Autodesk Fusion 360 part; units mm, degrees
(part 3 of 5)
sketch "Sketch6 (3)" plane through (0, 18.9, 0) normal (0, -1, 0) x (1, 0, 0) in component "main-switchbody (3)"
  line L0 (13.95, 0) -> (16.95, 0)
  line L1 (16.95, 0) -> (16.95, 6)
  line L2 (16.95, 6) -> (13.95, 6)
  line L3 (13.95, 6) -> (13.95, 0)
  line L4 (13.95, 6) -> (13.95, 4.5) construction
  line L5 (16.95, 6) -> (16.95, 4.5) construction
  arc A0 (16.95, 4.5) -> (13.95, 4.5) centre (15.45, 4.5) ccw
  constraint coincident L2.end L3.start
  constraint coincident L3 L4.end
  constraint perpendicular L2 L4
  constraint coincident L1.end L2.start
  constraint coincident L1 L5.end
  constraint perpendicular L2 L5
  constraint tangent L2 A0
extrude "Extrude10''" cut sketch "Sketch6 (3)" against normal blind 1.1 contours L2 L3 A0 | L1 L2 A0 bodies 24 in component "main-switchbody (3)"
sketch "Sketch7 (3)" plane through (0, 0, 4) normal (0, 0, 1) x (-1, 0, 0) in component "main-switchbody (3)"
  line L0 (-3.05, -16.95) -> (-16.95, -16.95)
  line L1 (-16.95, -16.95) -> (-16.95, -3.05)
  line L2 (-16.95, -3.05) -> (-3.05, -3.05)
  line L3 (-3.05, -3.05) -> (-3.05, -16.95)
  line L4 (-6.05, -20) -> (-6.05, -18.9)
  line L5 (-6.05, -18.9) -> (-3.05, -18.9)
  line L6 (-3.05, -18.9) -> (-3.05, -20)
  line L7 (-3.05, -20) -> (0, -20)
  line L8 (0, -20) -> (0, 0)
  line L9 (0, 0) -> (-3.05, 0)
  line L10 (-3.05, 0) -> (-3.05, -1.1)
  line L11 (-3.05, -1.1) -> (-6.05, -1.1)
  line L12 (-6.05, -1.1) -> (-6.05, 0)
  line L13 (-6.05, 0) -> (-13.95, 0)
  line L14 (-13.95, 0) -> (-13.95, -1.1)
  line L15 (-13.95, -1.1) -> (-16.95, -1.1)
  line L16 (-16.95, -1.1) -> (-16.95, 0)
  line L17 (-16.95, 0) -> (-20, 0)
  line L18 (-20, 0) -> (-20, -20)
  line L19 (-20, -20) -> (-16.95, -20)
  line L20 (-16.95, -20) -> (-16.95, -18.9)
  line L21 (-16.95, -18.9) -> (-13.95, -18.9)
  line L22 (-13.95, -18.9) -> (-13.95, -20)
  line L23 (-13.95, -20) -> (-6.05, -20)
  line L24 (-20, -10) -> (-20, -11.5) construction
  line L25 (-20, -10) -> (-20, -8.5) construction
  line L26 (-20, -8.5) -> (-19, -8.5) construction
  line L27 (-19, -8.5) -> (-19, -11.5) construction
  line L28 (-19, -11.5) -> (-20, -11.5) construction
  line L29 (-20, -11.5) -> (-21, -11.5) construction
  line L30 (-21, -11.5) -> (-21, -8.5) construction
  line L31 (-21, -8.5) -> (-20, -8.5) construction
  line L32 (-19, -11.5) -> (-21, -11.5)
  line L33 (-21, -11.5) -> (-21, -8.5)
  line L34 (-21, -8.5) -> (-19, -8.5)
  line L35 (-19, -8.5) -> (-19, -11.5)
  dimension "d41_6" = 1.5
  dimension "d42_6" = 1
  constraint midpoint L18 L24.start
  constraint parallel L18 L24
  constraint coincident L18 L25.end
  constraint parallel L18 L25
  constraint perpendicular L25 L26
  constraint perpendicular L26 L27
  constraint perpendicular L24 L29
  constraint perpendicular L29 L30
  constraint horizontal L32
  constraint vertical L33
  constraint horizontal L34
  constraint vertical L35
  measures "d41_6" distance of L24.start L24.end
  measures "d42_6" distance of L24.end L29.end
extrude "Extrude11''" add sketch "Sketch7 (3)" along normal blind 3 contours L18 L32 L33 L34 | L18 L32 L34 L35 bodies 20 in component "main-switchbody (3)"
extrude "Extrude12''" add 1 faces at (20, 8.5, 6) along direction (0, -1, 0) blind 0.5 on bodies 20 bodies 20 in component "main-switchbody (3)"
extrude "Extrude13''" add 1 faces at (20, 11.5, 6) along direction (0, 1, 0) blind 0.5 on bodies 20 bodies 20 in component "main-switchbody (3)"
extrude "Extrude14''" add 1 faces at (20.3333, 10.6667, 7) along direction (0, 0, 1) blind 0.75 on bodies 20 bodies 20 in component "main-switchbody (3)"
sketch "Sketch8 (3)" plane through (0, 0, 4) normal (0, 0, -1) x (1, 0, 0) in component "main-switchbody (3)"
  line L0 (20, -8) -> (20, -12)
  line L1 (20, -12) -> (21, -12)
  line L2 (21, -12) -> (21, -8)
  line L3 (21, -8) -> (20, -8)
  line L4 (20, -12) -> (20, -8)
  constraint coincident L0.end L1.start
  constraint coincident L0.start L3.end
extrude "Extrude15''" add sketch "Sketch8 (3)" along normal blind 2 bodies 20 in component "main-switchbody (3)"
sketch "Sketch9 (5)" plane through (19, 0, 0) normal (-1, 0, 0) x (0, -1, 0) in component "main-switchbody (3)"
  line L0 (-12, 4) -> (-8, 4)
  line L1 (-8, 4) -> (-8, 7.75)
  line L2 (-8, 7.75) -> (-12, 7.75)
  line L3 (-12, 7.75) -> (-12, 4)
  line L4 (-12, 7.75) -> (-12, 5.75) construction
  line L5 (-12, 5.75) -> (-8, 5.75) construction
  line L6 (-12, 7.75) -> (-8, 7.75)
  line L7 (-8, 7.75) -> (-8, 5.75)
  line L8 (-8, 5.75) -> (-12, 5.75)
  line L9 (-12, 5.75) -> (-12, 7.75)
  dimension "d53_6" = 2
  constraint coincident L2.end L3.start
  constraint perpendicular L2 L4
  constraint coincident L1 L5.end
  constraint perpendicular L1 L5
  constraint horizontal L6
  constraint vertical L7
  constraint horizontal L8
  constraint vertical L9
  measures "d53_6" distance of L2.end L4.end
extrude "Extrude16''" add sketch "Sketch9 (5)" along normal blind 0.5 contours L1 L2 L3 L6 L7 L8 L9 bodies 20 in component "main-switchbody (3)"
extrude "Extrude17''" cut 1 faces at (2.1, 9.3333, 6.9167) along direction (-1, 0, 0) blind 0.3 on bodies 19 bodies 19 in component "main-switchbody (3)"
extrude "Extrude18''" cut sketch "Sketch1 (13)" along normal blind 2.7 contours L44 L84 L85 L86 L87 bodies 20 in component "main-switchbody (3)"
extrude "Extrude19''" cut sketch "Sketch1 (13)" along normal blind 2.7 contours L46 L80 L81 L82 L83 bodies 20 in component "main-switchbody (3)"
extrude "Extrude20''" add sketch "Sketch1 (13)" against normal blind 0.2 contours L39 L40 L41 L42 L47 L48 L50 L51 L52 L54 L56 L57 L58 L60 L61 L62 L63 L64 L65 L66 L67 L68 | L39 L59 L60 L61 L62 | L42 L63 L64 L65 L66 L67 L68 | L39 L55 L56 L57 L58 | L41 L47 L48 L49 L50 | L41 L51 L52 L53 L54 bodies 19 20 21 22 23 24 in component "main-switchbody (3)"
fillet "Fillet1''" radius 1 2 edges at (21, 10, 7.75) (-0.9, 10, 7.5) on bodies 19 20 in component "main-switchbody (3)"
extrude "Extrude21''" add 1 faces at (2.8833, 9.1667, 2.7) along direction (0, 0, -1) blind 2.9 on bodies 19 bodies 19 in component "main-switchbody (3)"
extrude "Extrude22''" add 1 faces at (17.1167, 10.8333, 2.7) along direction (0, 0, -1) blind 2.9 on bodies 19 bodies 19 in component "main-switchbody (3)"
sketch "Sketch10 (3)" plane through (0, 0, 4) normal (0, 0, 1) x (-1, 0, 0) in component "main-switchbody (3)"
  line L0 (-3.05, -16.95) -> (-16.95, -16.95)
  line L1 (-16.95, -16.95) -> (-16.95, -3.05)
  line L2 (-16.95, -3.05) -> (-3.05, -3.05)
  line L3 (-3.05, -3.05) -> (-3.05, -16.95)
  line L4 (0, -12) -> (-1.1, -12)
  line L5 (-1.1, -12) -> (-1.1, -8)
  line L6 (-1.1, -8) -> (0, -8)
  line L7 (0, -8) -> (0, 0)
  line L8 (0, 0) -> (-3.05, 0)
  line L9 (-3.05, 0) -> (-3.05, -1.1)
  line L10 (-3.05, -1.1) -> (-6.05, -1.1)
  line L11 (-6.05, -1.1) -> (-6.05, 0)
  line L12 (-6.05, 0) -> (-13.95, 0)
  line L13 (-13.95, 0) -> (-13.95, -1.1)
  line L14 (-13.95, -1.1) -> (-16.95, -1.1)
  line L15 (-16.95, -1.1) -> (-16.95, 0)
  line L16 (-16.95, 0) -> (-20, 0)
  line L17 (-20, 0) -> (-20, -8)
  line L18 (-20, -8) -> (-19, -8)
  line L19 (-19, -8) -> (-19, -12)
  line L20 (-19, -12) -> (-20, -12)
  line L21 (-20, -12) -> (-20, -20)
  line L22 (-20, -20) -> (-16.95, -20)
  line L23 (-16.95, -20) -> (-16.95, -18.9)
  line L24 (-16.95, -18.9) -> (-13.95, -18.9)
  line L25 (-13.95, -18.9) -> (-13.95, -20)
  line L26 (-13.95, -20) -> (-6.05, -20)
  line L27 (-6.05, -20) -> (-6.05, -18.9)
  line L28 (-6.05, -18.9) -> (-3.05, -18.9)
  line L29 (-3.05, -18.9) -> (-3.05, -20)
  line L30 (-3.05, -20) -> (0, -20)
  line L31 (0, -20) -> (0, -12)
  line L32 (-3.05, -10) -> (-3.05, -12.5) construction
  line L33 (-3.05, -12.5) -> (-3.05, -7.5) construction
  line L34 (-3.05, -7.5) -> (-2.55, -7.5) construction
  line L35 (-2.55, -7.5) -> (-3.05, -7.5) construction
  line L36 (-3.05, -7.5) -> (-3.05, -12.5) construction
  line L37 (-3.05, -12.5) -> (-2.55, -12.5) construction
  line L38 (-2.55, -12.5) -> (-2.55, -7.5) construction
  line L39 (-3.05, -12.5) -> (-16.95, -12.5) construction
  line L40 (-16.95, -12.5) -> (-16.95, -7.5) construction
  line L41 (-16.95, -7.5) -> (-17.45, -7.5) construction
  line L42 (-17.45, -7.5) -> (-16.95, -7.5) construction
  line L43 (-16.95, -7.5) -> (-16.95, -12.5) construction
  line L44 (-16.95, -12.5) -> (-17.45, -12.5) construction
  line L45 (-17.45, -12.5) -> (-17.45, -7.5) construction
  line L46 (-16.95, -12.5) -> (-17.45, -12.5)
  line L47 (-17.45, -12.5) -> (-17.45, -7.5)
  line L48 (-17.45, -7.5) -> (-16.95, -7.5)
  line L49 (-16.95, -7.5) -> (-16.95, -12.5)
  line L50 (-2.55, -12.5) -> (-3.05, -12.5)
  line L51 (-3.05, -12.5) -> (-3.05, -7.5)
  line L52 (-3.05, -7.5) -> (-2.55, -7.5)
  line L53 (-2.55, -7.5) -> (-2.55, -12.5)
  dimension "d75_3" = 5
  dimension "d76_3" = 0.5
  dimension "d77_3" = 0.5
  constraint midpoint L3 L32.start
  constraint coincident L3 L32.end
  constraint perpendicular L0 L32
  constraint parallel L3 L33
  constraint perpendicular L33 L34
  constraint horizontal L35
  constraint vertical L36
  constraint horizontal L37
  constraint vertical L38
  constraint coincident L1 L39.end
  constraint perpendicular L1 L39
  constraint coincident L1 L40.end
  constraint perpendicular L39 L40
  constraint perpendicular L40 L41
  constraint horizontal L42
  constraint vertical L43
  constraint horizontal L44
  constraint vertical L45
  constraint horizontal L46
  constraint vertical L47
  constraint horizontal L48
  constraint vertical L49
  constraint horizontal L50
  constraint vertical L51
  constraint horizontal L52
  constraint vertical L53
  measures "d75_3" distance of L32.end L33.end
  measures "d76_3" distance of L33.end L34.end
  measures "d77_3" distance of L40.end L41.end
extrude "Extrude23''" cut sketch "Sketch10 (3)" against normal blind 2.9 contours L3 L50 L51 L52 L53 | L1 L46 L47 L48 L49 bodies 19 in component "main-switchbody (3)"
extrude "Extrude24''" cut 2 faces at (4.8122, 18.9, 5.1079) (15.1626, 18.9, 5.4316) along direction (0, 1, 0) blind 0.25 on bodies 19 bodies 19 in component "main-switchbody (3)"
extrude "Extrude25''" cut 2 faces at (4.2822, 1.1, 5.1824) (15.2673, 1.1, 4.9654) along direction (0, -1, 0) blind 0.25 on bodies 19 bodies 19 in component "main-switchbody (3)"
extrude "Extrude26''" add 1 faces at (1.0167, 12.3167, -0.2) along direction (0, 0, -1) blind 1 on bodies 19 bodies 19 in component "main-switchbody (3)"
extrude "Extrude27''" cut 1 faces at (1.0167, 12.3167, -1.2) along direction (0, 0, 1) blind 0.2 on bodies 19 bodies 19 in component "main-switchbody (3)"
extrude "Extrude28''" cut 2 faces at (17.1167, 10.8333, 1.1) (2.8833, 9.1667, 1.1) along direction (0, 0, -1) blind 0.8 on bodies 19 bodies 19 in component "main-switchbody (3)"
extrude "Extrude29''" cut 1 faces at (18.8333, 9.3333, 5.75) along direction (0, 0, 1) blind 0.2 on bodies 19 bodies 19 in component "main-switchbody (3)"
extrude "Extrude30''" cut 1 faces at (1.3333, 10.6667, 5.75) along direction (0, 0, 1) blind 0.2 on bodies 19 bodies 19 in component "main-switchbody (3)"
sketch "Sketch1 (14)" plane through (0, 0, 0.0152) normal (0, 0, -1) x (1, 0, 0) in component "mxledbit-switchbody v10 (3)"
  line L0 (4.5419, -16.2374) -> (4.5419, -2.3374)
  line L1 (4.5419, -2.3374) -> (18.4419, -2.3374)
  line L2 (18.4419, -2.3374) -> (18.4419, -16.2374)
  line L3 (18.4419, -16.2374) -> (4.5419, -16.2374)
  line L4 (1.4919, -19.2874) -> (21.4919, -19.2874)
  line L5 (21.4919, -19.2874) -> (21.4919, 0.7126)
  line L6 (21.4919, 0.7126) -> (1.4919, 0.7126)
  line L7 (1.4919, 0.7126) -> (1.4919, -19.2874)
ref_plane "WorkPlane1" through (5, 36.1899, 12.0831) normal (0, -0.996195, 0.087156) x (1, 0, 0) in component "wheel (2)"
sketch "Sketch2 (11)" plane through (5, 36.1899, 12.0831) normal (0, -0.996195, 0.087156) x (1, 0, 0) in component "wheel (2)"
  circle A0 centre (0, 0) radius 85
  dimension "d64_3" = 170
  constraint coincident A0.centre origin
  measures "d64_3" diameter of A0
component_pattern "component pattern''" in component "Middle"
sketch "Sketch2 (12)" plane through (0, 32.8735, -2.8761) normal (0, -0.996195, 0.087156) x (1, 0, 0) in component "IND-Sketch (2)"
  circle A0 centre (5, 15.1913) radius 85
  line L0 (5, 15.1913) -> (5, -69.8087) construction
  line L1 (5, -69.8087) -> (-12, -69.8087) construction
  line L2 (-12, -69.8087) -> (22, -69.8087)
  line L3 (22, -69.8087) -> (22, 15.1913)
  line L4 (22, 15.1913) -> (-12, 15.1913)
  line L5 (-12, 15.1913) -> (-12, -69.8087)
  dimension "d69_3" = 85
  dimension "d70_3" = 17
  dimension "d71_3" = 34
  dimension "d72_3" = 85
  constraint coincident A0.centre L0.start
  constraint vertical L0
  constraint perpendicular L0 L1
  constraint horizontal L2
  constraint vertical L3
  constraint horizontal L4
  constraint vertical L5
  measures "d69_3" distance of A0.centre L0.end
  measures "d70_3" distance of L0.end L1.end
  measures "d71_3" distance of L1.end L2.end
  measures "d72_3" distance of L1.end L4.end
sketch "Sketch9 (6)" plane through (5, 41.9534, 55.6343) normal (0, 0.573576, 0.819152) x (-1, 0, 0) in component "IND-Sketch (2)"
  line L0 (-45, -9.823) -> (5, -9.823) construction
  line L1 (-20, -9.823) -> (5, -9.823) construction
  line L2 (-20, -9.823) -> (-45, -9.823) construction
  circle A0 centre (-20, -9.823) radius 75 construction
  point P0 (-20, -9.823)
  point P1 (-45, -9.823)
  point P2 (5, -9.823)
  point P3 (5, -9.823)
  point P4 (-45, -9.823)
  dimension "d38_3" = 34
  dimension "d39_3" = 17
  dimension "d40_3" = 17
  dimension "d41_3" = 170
  constraint coincident P4 P1
  constraint horizontal L0
  constraint coincident P0 L1.start
  constraint parallel L0 L1
  constraint parallel L0 L2
sketch "Sketch1 (15)" plane through (0, 54.7581, -45.9475) normal (0, -0.766044, 0.642788) x (1, 0, 0) in component "IND-Sketch (2)"
  line L0 (-1.3269, 70.632) -> (-1.3269, 84.532)
  line L1 (-1.3269, 84.532) -> (12.5731, 84.532)
  line L2 (12.5731, 84.532) -> (12.5731, 70.632)
  line L3 (12.5731, 70.632) -> (-1.3269, 70.632)
  line L4 (-4.3769, 67.582) -> (15.6231, 67.582)
  line L5 (15.6231, 67.582) -> (15.6231, 87.582)
  line L6 (15.6231, 87.582) -> (-4.3769, 87.582)
  line L7 (-4.3769, 87.582) -> (-4.3769, 67.582)
  line L8 (-4.3769, 77.582) -> (15.6231, 77.582) construction
  line L9 (5.6231, 87.582) -> (5.6231, 67.582) construction
  point P0 (5.6231, 77.582)
  constraint midpoint L7 L8.start
  constraint midpoint L5 L8.end
  constraint midpoint L6 L9.start
  constraint midpoint L4 L9.end
  constraint midpoint L8 P0
ref_plane "WorkPlane2" through (0, 49, 0) normal (0, 1, 0) x (0, 0, 1) in component "IND-Sketch (3)"
sketch "IND-originXY (4)" plane through (0, 0, 0) normal (0, 0, 1) x (1, 0, 0) in component "IND-Sketch (3)"
  line L0 (0, 0) -> (0, 16) construction
  line L1 (0, 16) -> (16, 16) construction
  line L2 (16, 16) -> (16, -33) construction
  line L3 (16, -33) -> (-33, -33) construction
  line L4 (0, 16) -> (24.5, 16) construction
  point P0 (24.5, 16)
  dimension "d20_7" = 16
  dimension "d21_7" = 16
  dimension "d29_7" = 49
  dimension "d30_7" = 49
  dimension "d34_7" = 24.5
  constraint coincident L0.start origin
  constraint vertical L0
  constraint perpendicular L0 L1
  constraint perpendicular L1 L2
  constraint perpendicular L0 L3
  constraint perpendicular L0 L4
  constraint coincident P0 L4.end
  measures "d20_7" distance of L0.start L0.end
  measures "d21_7" distance of L0.end L1.end
  measures "d29_7" distance of L1.end L2.end
  measures "d30_7" distance of L2.end L3.end
  measures "d34_7" distance of L0.end P0
sketch "IND-originXZ (4)" plane through (0, 49, 0) normal (0, 1, 0) x (1, 0, 0) in component "IND-Sketch (3)"
  line L0 (0, 0) -> (16, 0) construction
  line L1 (10, 0) -> (10, -10) construction
  line L2 (10, -10) -> (0, -10) construction
  line L3 (0, -10) -> (0, 0) construction
  line L4 (10, -10) -> (5, -10) construction
  line L5 (0, -10) -> (5, -10) construction
  line L6 (0, -10) -> (5, -10) construction
  point P0 (16, 0)
  point P1 (0, -10)
  point P2 (10, -10)
  point P3 (24.5, 0)
  point P4 (5, -10)
  dimension "d26_7" = 10
  dimension "d27_7" = 49
  dimension "d28_7" = 49
  dimension "d36_7" = 24.5
  dimension "d37_7" = 24.5
  constraint coincident P0 L1.start
  constraint perpendicular L0 L1
  constraint perpendicular L1 L2
  constraint coincident L0.start L3.end
  constraint coincident P1 L2.end
  constraint coincident P2 L1.end
  constraint midpoint L2 P4
  constraint perpendicular L1 L4
  constraint parallel L4 L6
  measures "d26_7" distance of L1.start P2
ref_plane "WorkPlane3" through (5, 49, 10) normal (0, 1, 0) x (-1, 0, 0) in component "IND-Sketch (3)"
sketch "IND-path (4)" plane through (5, 49, 10) normal (0, 1, 0) x (-1, 0, 0) in component "IND-Sketch (3)"
  line L0 (-5, 0) -> (5, 0) construction
  line L1 (5, 0) -> (-5, 0) construction
  circle A0 centre (0, 0) radius 75 construction
  line L2 (0, 0) -> (24.5, 0) construction
  line L3 (0, 0) -> (-24.5, 0) construction
  line L4 (0, 0) -> (0, -75) construction
  line L5 (0, -75) -> (6.95, -75) construction
  line L6 (0, -75) -> (-6.95, -75) construction
  point P0 (-5, 0)
  point P1 (5, 0)
  point P2 (0, -75)
  dimension "d32_7" = 150
  dimension "d33_7" = 24.5
  dimension "d35_7" = 24.5
  dimension "d42_7" = 75
  dimension "d43_7" = 6.95
  dimension "d44_7" = 6.95
  dimension "d67_7" = 90
  constraint coincident P1 L0.end
  constraint coincident P0 L0.start
  constraint coincident A0.centre L2.start
  constraint parallel L1 L2
  constraint parallel L0 L3
  constraint coincident P2 L4.end
  constraint perpendicular L4 L5
  constraint perpendicular L4 L6
  measures "d32_7" diameter of A0
  measures "d33_7" distance of A0.centre L2.end
  measures "d35_7" distance of A0.centre L3.end
  measures "d42_7" distance of A0.centre P2
  measures "d43_7" distance of P2 L5.end
  measures "d44_7" distance of P2 L6.end
  measures "d67_7" angle of L2 L4
sketch "Sketch1 (16)" plane through (5, 49, 10) normal (0, 1, 0) x (-1, 0, 0) in component "wheel (3)"
  circle A0 centre (0, 0) radius 75
  line L0 (0, -75) -> (6.95, -75)
  line L1 (0, -75) -> (-6.95, -75)
  line L2 (0, -75) -> (0, 75) construction
  line L3 (0, 0) -> (75, 0) construction
  circle A1 centre (0, 0) radius 75
  point P0 (0, -75)
  dimension "d45_7" = 150
  dimension "d46_7" = 75
  dimension "d47_7" = 150
  constraint coincident P0 L0.start
  constraint perpendicular L0 L2
  constraint coincident A0.centre L3.start
  constraint perpendicular L2 L3
  measures "d45_7" distance of P0 L2.end
  measures "d46_7" distance of A0.centre L3.end
  measures "d47_7" diameter of A1
extrude "Extrude1'''''''''" add sketch "Sketch1 (16)" along normal blind 4 separate body makes body 25 in component "wheel (3)"
ref_plane "WorkPlane1" through (5, 70.3992, -65) normal (0, 0, -1) x (1, 0, 0) in component "plug (3)"
sketch "Sketch1 (17)" plane through (5, 31.3992, -65) normal (0, 0, -1) x (1, 0, 0) in component "plug (3)"
  line L0 (-75, -21.6008) -> (75, -21.6008)
  line L1 (-75, -21.6008) -> (75, -21.6008)
  line L2 (-75, -17.6008) -> (75, -17.6008)
  line L3 (-75, -17.6008) -> (75, -17.6008)
  line L4 (0, -17.6008) -> (0, -21.6008) construction
  line L5 (0, -17.6008) -> (-6.95, -17.6008) construction
  line L6 (0, -17.6008) -> (6.95, -17.6008) construction
  line L7 (6.95, -17.6008) -> (6.95, -21.6008) construction
  line L8 (-6.95, -17.6008) -> (-6.95, -21.6008) construction
  line L9 (-6.95, -21.6008) -> (6.95, -21.6008) construction
  line L10 (6.95, -21.6008) -> (-6.95, -21.6008)
  line L11 (-6.95, -21.6008) -> (-6.95, -17.6008)
  line L12 (-6.95, -17.6008) -> (6.95, -17.6008)
  line L13 (6.95, -17.6008) -> (6.95, -21.6008)
  point P0 (0, -17.6008)
  dimension "d51_7" = 6.95
  dimension "d52_7" = 6.95
  constraint coincident P0 L4.start
  constraint midpoint L1 L4.end
  constraint perpendicular L4 L5
  constraint perpendicular L4 L6
  constraint coincident L1 L7.end
  constraint perpendicular L1 L7
  constraint coincident L0 L8.end
  constraint perpendicular L0 L8
  constraint horizontal L10
  constraint vertical L11
  constraint horizontal L12
  constraint vertical L13
  measures "d51_7" distance of P0 L5.end
  measures "d52_7" distance of P0 L6.end
extrude "Extrude1''''''''''" add sketch "Sketch1 (17)" along normal blind 4 separate body makes body 26 in component "plug (3)"
sketch "Sketch2 (13)" plane through (0, 0, -65) normal (0, 0, 1) x (1, 0, 0) in component "plug (3)"
  line L0 (-1.95, 49) -> (11.95, 49)
  line L1 (11.95, 49) -> (11.95, 53)
  line L2 (11.95, 53) -> (-1.95, 53)
  line L3 (-1.95, 53) -> (-1.95, 49)
extrude "Extrude2''''''" add 1 faces at (2.6833, 53, -67.6667) along direction (0, 1, 0) blind 4.95 on bodies 26 bodies 26 in component "plug (3)"
extrude "Extrude3''''''" add 1 faces at (2.6833, 49, -67.6667) along direction (0, -1, 0) blind 4.95 on bodies 26 bodies 26 in component "plug (3)"
sketch "Sketch1 (18)" plane through (0, 0, 0) normal (0, 0, 1) x (1, 0, 0) in component "main-switchbody (5)"
  line L0 (0, 0) -> (0, 20) construction
  line L1 (0, 20) -> (20, 20) construction
  line L2 (20, 20) -> (20, 0) construction
  line L3 (20, 0) -> (0, 0) construction
  line L4 (0, 0) -> (20, 20) construction
  line L5 (20, 0) -> (0, 20) construction
  line L6 (10, 0) -> (18.9, 0) construction
  line L7 (10, 10) -> (18.9, 10) construction
  line L8 (18.9, 10) -> (18.9, 18.9) construction
  line L9 (18.9, 18.9) -> (1.1, 18.9) construction
  line L10 (1.1, 18.9) -> (1.1, 1.1) construction
  line L11 (1.1, 1.1) -> (18.9, 1.1) construction
  line L12 (18.9, 1.1) -> (18.9, 18.9) construction
  line L13 (10, 10) -> (3.05, 10) construction
  line L14 (3.05, 10) -> (3.05, 16.95) construction
  line L15 (3.05, 16.95) -> (16.95, 16.95) construction
  line L16 (16.95, 16.95) -> (16.95, 3.05) construction
  line L17 (16.95, 3.05) -> (3.05, 3.05) construction
  line L18 (3.05, 3.05) -> (3.05, 16.95) construction
  line L19 (3.05, 3.05) -> (0, 3.05) construction
  line L20 (3.05, 3.05) -> (3.05, 0) construction
  line L21 (16.95, 3.05) -> (20, 3.05) construction
  line L22 (16.95, 16.95) -> (20, 16.95) construction
  line L23 (16.95, 16.95) -> (16.95, 20) construction
  line L24 (3.05, 16.95) -> (3.05, 20) construction
  line L25 (3.05, 16.95) -> (0, 16.95) construction
  line L26 (3.05, 18.9) -> (6.05, 18.9) construction
  line L27 (6.05, 18.9) -> (6.05, 20) construction
  line L28 (16.95, 18.9) -> (13.95, 18.9) construction
  line L29 (13.95, 18.9) -> (13.95, 20) construction
  line L30 (16.95, 3.05) -> (16.95, 0) construction
  line L31 (16.95, 1.1) -> (13.95, 1.1) construction
  line L32 (13.95, 1.1) -> (13.95, 0) construction
  line L33 (3.05, 1.1) -> (6.05, 1.1) construction
  line L34 (6.05, 1.1) -> (6.05, 0) construction
  line L35 (0, 20) -> (20, 20) construction
  line L36 (20, 20) -> (20, 0) construction
  line L37 (20, 0) -> (0, 0) construction
  line L38 (0, 0) -> (0, 20) construction
  line L39 (0, 20) -> (20, 20)
  line L40 (20, 20) -> (20, 0)
  line L41 (20, 0) -> (0, 0)
  line L42 (0, 0) -> (0, 20)
  line L43 (16.95, 3.05) -> (3.05, 3.05)
  line L44 (3.05, 3.05) -> (3.05, 16.95)
  line L45 (3.05, 16.95) -> (16.95, 16.95)
  line L46 (16.95, 16.95) -> (16.95, 3.05)
  line L47 (3.05, 1.1) -> (6.05, 1.1)
  line L48 (6.05, 1.1) -> (6.05, 0)
  line L49 (6.05, 0) -> (3.05, 0)
  line L50 (3.05, 0) -> (3.05, 1.1)
  line L51 (13.95, 1.1) -> (16.95, 1.1)
  line L52 (16.95, 1.1) -> (16.95, 0)
  line L53 (16.95, 0) -> (13.95, 0)
  line L54 (13.95, 0) -> (13.95, 1.1)
  line L55 (13.95, 20) -> (16.95, 20)
  line L56 (16.95, 20) -> (16.95, 18.9)
  line L57 (16.95, 18.9) -> (13.95, 18.9)
  line L58 (13.95, 18.9) -> (13.95, 20)
  line L59 (3.05, 20) -> (6.05, 20)
  line L60 (6.05, 20) -> (6.05, 18.9)
  line L61 (6.05, 18.9) -> (3.05, 18.9)
  line L62 (3.05, 18.9) -> (3.05, 20)
  line L63 (1.1, 10) -> (1.1, 12)
  line L64 (1.1, 10) -> (1.1, 8)
  line L65 (1.1, 8) -> (-1.9, 8)
  line L66 (-1.9, 8) -> (1.1, 8)
  line L67 (1.1, 8) -> (1.1, 12)
  line L68 (1.1, 12) -> (-1.9, 12)
  line L69 (-1.9, 12) -> (-1.9, 8)
  line L70 (3.05, 10) -> (3.05, 7.5) construction
  line L71 (3.05, 7.5) -> (2.55, 7.5) construction
  line L72 (2.55, 7.5) -> (2.55, 12.5) construction
  line L73 (2.55, 12.5) -> (3.05, 12.5085) construction
  line L74 (3.05, 12.5085) -> (3.05, 7.5) construction
  line L75 (2.55, 12.5) -> (16.95, 12.5) construction
  line L76 (16.95, 12.5) -> (17.45, 12.5) construction
  line L77 (17.45, 12.5) -> (17.45, 7.5) construction
  line L78 (17.45, 7.5) -> (16.95, 7.5) construction
  line L79 (16.95, 7.5) -> (16.95, 12.5) construction
  line L80 (17.45, 7.5) -> (16.95, 7.5)
  line L81 (16.95, 7.5) -> (16.95, 12.5)
  line L82 (16.95, 12.5) -> (17.45, 12.5)
  line L83 (17.45, 12.5) -> (17.45, 7.5)
  line L84 (3.05, 7.5) -> (2.55, 7.5)
  line L85 (2.55, 7.5) -> (2.55, 12.5)
  line L86 (2.55, 12.5) -> (3.05, 12.5)
  line L87 (3.05, 12.5) -> (3.05, 7.5)
  dimension "d1_5" = 20
  dimension "d2_5" = 20
  dimension "d3_5" = 8.9
  dimension "d4_5" = 8.9
  dimension "d5_5" = 8.9
  dimension "d6_5" = 17.8
  dimension "d7_5" = 17.8
  dimension "d8_5" = 6.95
  dimension "d9_5" = 6.95
  dimension "d10_5" = 13.9
  dimension "d11_5" = 13.9
  dimension "d12_5" = 13.9
  dimension "d13_5" = 3
  dimension "d14_5" = 3
  dimension "d15_5" = 3
  dimension "d16_5" = 3
  dimension "d21_9" = 3
  dimension "d58_9" = 2.5
  dimension "d59_9" = 0.5
  dimension "d60_9" = 5
  dimension "d61_9" = 0.5
  dimension "d62_9" = 5
  constraint coincident L0.start L3.end
  constraint vertical L0
  constraint perpendicular L0 L1
  constraint perpendicular L1 L2
  constraint perpendicular L0 L3
  constraint midpoint L3 L6.start
  constraint parallel L3 L6
  constraint midpoint L4 L7.start
  constraint parallel L6 L7
  constraint perpendicular L7 L8
  constraint perpendicular L8 L9
  constraint perpendicular L9 L10
  constraint coincident L5 L11.end
  constraint perpendicular L10 L11
  constraint perpendicular L12 L13
  constraint perpendicular L13 L14
  constraint perpendicular L14 L15
  constraint perpendicular L7 L16
  constraint perpendicular L16 L17
  constraint coincident L0 L19.end
  constraint perpendicular L0 L19
  constraint coincident L3 L20.end
  constraint perpendicular L3 L20
  constraint coincident L2 L21.end
  constraint perpendicular L2 L21
  constraint coincident L2 L22.end
  constraint perpendicular L2 L22
  constraint coincident L1 L23.end
  constraint perpendicular L1 L23
  constraint coincident L1 L24.end
  constraint perpendicular L1 L24
  constraint coincident L0 L25.end
  constraint perpendicular L0 L25
  constraint coincident L24 L26.start
  constraint coincident L9 L26.start
  constraint coincident L9 L26.end
  constraint coincident L1 L27.end
  constraint perpendicular L1 L27
  constraint coincident L9 L28.start
  constraint coincident L23 L28.start
  constraint perpendicular L23 L28
  constraint coincident L1 L29.end
  constraint perpendicular L1 L29
  constraint coincident L6 L30.end
  constraint coincident L30 L31.start
  constraint coincident L11 L31.start
  constraint perpendicular L30 L31
  constraint coincident L6 L32.end
  constraint coincident L11 L33.start
  constraint coincident L20 L33.start
  constraint perpendicular L20 L33
  constraint coincident L3 L34.end
  constraint perpendicular L3 L34
  constraint horizontal L35
  constraint vertical L36
  constraint horizontal L37
  constraint vertical L38
  constraint horizontal L39
  constraint vertical L40
  constraint horizontal L41
  constraint vertical L42
  constraint horizontal L43
  constraint vertical L44
  constraint horizontal L45
  constraint vertical L46
  constraint horizontal L47
  constraint vertical L48
  constraint horizontal L49
  constraint vertical L50
  constraint horizontal L51
  constraint vertical L52
  constraint horizontal L53
  constraint vertical L54
  constraint horizontal L55
  constraint vertical L56
  constraint horizontal L57
  constraint vertical L58
  constraint horizontal L59
  constraint vertical L60
  constraint horizontal L61
  constraint vertical L62
  constraint midpoint L10 L63.start
  constraint coincident L10 L63.end
  constraint parallel L10 L63
  constraint coincident L10 L64.end
  constraint perpendicular L0 L65
  constraint horizontal L66
  constraint vertical L67
  constraint horizontal L68
  constraint vertical L69
  constraint perpendicular L13 L70
  constraint perpendicular L70 L71
  constraint perpendicular L71 L72
  constraint coincident L14 L73.end
  constraint perpendicular L71 L74
  constraint coincident L16 L75.end
  constraint perpendicular L16 L75
  constraint perpendicular L16 L76
  constraint perpendicular L76 L77
  constraint coincident L16 L78.end
  constraint perpendicular L16 L78
  constraint horizontal L80
  constraint vertical L81
  constraint horizontal L82
  constraint vertical L83
  constraint horizontal L84
  constraint vertical L85
  constraint horizontal L86
  constraint vertical L87
  measures "d1_5" distance of L0.start L0.end
  measures "d2_5" distance of L0.end L1.end
  measures "d3_5" distance of L6.start L6.end
  measures "d4_5" distance of L7.start L7.end
  measures "d5_5" distance of L7.end L8.end
  measures "d6_5" distance of L8.end L9.end
  measures "d7_5" distance of L9.end L10.end
  measures "d8_5" distance of L7.start L13.end
  measures "d9_5" distance of L13.end L14.end
  measures "d10_5" distance of L14.end L15.end
  measures "d11_5" distance of L15.end L16.end
  measures "d12_5" distance of L16.end L17.end
  measures "d13_5" distance of L26.start L26.end
  measures "d14_5" distance of L28.start L28.end
  measures "d15_5" distance of L31.start L31.end
  measures "d16_5" distance of L33.start L33.end
  measures "d21_9" distance of L64.end L65.end
  measures "d58_9" distance of L13.end L70.end
  measures "d59_9" distance of L70.end L71.end
  measures "d60_9" distance of L71.end L72.end
  measures "d61_9" distance of L75.end L76.end
  measures "d62_9" distance of L76.end L77.end
extrude "Extrude3'''''''" add sketch "Sketch1 (18)" along normal blind 7.5 separate body contours L42 L63 L64 L65 L66 L67 L68 | L42 L65 L66 L68 L69 makes body 27 in component "main-switchbody (5)"
extrude "Extrude2'''''''" add sketch "Sketch1 (18)" along normal blind 4 separate body contours L39 L40 L41 L42 L47 L48 L50 L51 L52 L54 L56 L57 L58 L60 L61 L62 L63 L64 L65 L66 L67 L68 | L42 L63 L64 L65 L66 L67 L68 | L46 L80 L81 L82 L83 | L44 L84 L85 L86 L87 makes body 28 in component "main-switchbody (5)"
extrude "Extrude1'''''''''''" add sketch "Sketch1 (18)" along normal blind 6 separate body contours L39 L59 L60 L61 L62 | L39 L55 L56 L57 L58 | L41 L47 L48 L49 L50 | L41 L51 L52 L53 L54 makes body 29 at (4.05, 1.1, 2) makes body 30 at (5.05, 20, 4) makes body 31 at (14.95, 1.1, 2) makes body 32 at (14.95, 20, 2) in component "main-switchbody (5)"
extrude "Extrude4'''" cut sketch "Sketch1 (18)" along normal blind 2 contours L42 L65 L66 L68 L69 bodies 27 in component "main-switchbody (5)"
sketch "Sketch2 (14)" plane through (1.1, 0, 0) normal (1, 0, 0) x (0, 1, 0) in component "main-switchbody (5)"
  line L0 (8, 0) -> (12, 0)
  line L1 (12, 0) -> (12, 7.5)
  line L2 (12, 7.5) -> (8, 7.5)
  line L3 (8, 7.5) -> (8, 0)
  line L4 (8, 7.5) -> (8, 4) construction
  line L5 (8, 4) -> (12, 4) construction
  line L6 (12, 4) -> (12, 7.5) construction
  line L7 (12, 7.5) -> (8, 7.5) construction
  line L8 (8, 7.5) -> (8, 5.75) construction
  line L9 (8, 5.75) -> (12, 5.75) construction
  line L10 (8, 7.5) -> (12, 7.5)
  line L11 (12, 7.5) -> (12, 5.75)
  line L12 (12, 5.75) -> (8, 5.75)
  line L13 (8, 5.75) -> (8, 7.5)
  dimension "d26_9" = 1.75
  constraint coincident L2.end L3.start
  constraint coincident L3 L4.end
  constraint perpendicular L2 L4
  constraint coincident L1 L5.end
  constraint perpendicular L1 L5
  constraint coincident L1.end L2.start
  constraint perpendicular L2 L6
  constraint perpendicular L5 L8
  constraint midpoint L6 L9.end
  constraint horizontal L10
  constraint vertical L11
  constraint horizontal L12
  constraint vertical L13
  measures "d26_9" distance of L2.end L8.end
extrude "Extrude5'''" add sketch "Sketch2 (14)" along normal blind 1 contours L1 L2 L3 L10 L11 L12 L13 bodies 27 in component "main-switchbody (5)"
extrude "Extrude6'''" cut 1 faces at (-1.9, 10.6667, 3.8333) along direction (1, 0, 0) blind 1 on bodies 27 bodies 27 in component "main-switchbody (5)"
sketch "Sketch3 (4)" plane through (0, 18.9, 0) normal (0, -1, 0) x (1, 0, 0) in component "main-switchbody (5)"
  line L0 (3.05, 0) -> (6.05, 0)
  line L1 (6.05, 0) -> (6.05, 6)
  line L2 (6.05, 6) -> (3.05, 6)
  line L3 (3.05, 6) -> (3.05, 0)
  line L4 (3.05, 6) -> (3.05, 4) construction
  line L5 (6.05, 4) -> (6.05, 6) construction
  line L6 (3.05, 6) -> (3.05, 4.5) construction
  line L7 (6.05, 6) -> (6.05, 4.5) construction
  arc A0 (6.05, 4.5) -> (3.05, 4.5) centre (4.55, 4.5) ccw construction
  arc A1 (6.05, 4.5) -> (3.05, 4.5) centre (4.55, 4.5) ccw
  dimension "d31_9" = 1.5
  dimension "d32_9" = 1.5
  constraint coincident L2.end L3.start
  constraint coincident L3 L4.end
  constraint perpendicular L2 L4
  constraint coincident L1 L5.start
  constraint coincident L1.end L2.start
  constraint perpendicular L2 L5
  constraint perpendicular L2 L6
  constraint perpendicular L2 L7
  constraint tangent L2 A0
  constraint tangent L2 A1
  measures "d31_9" distance of L2.end L6.end
  measures "d32_9" distance of L1.end L7.end
extrude "Extrude7'''" cut sketch "Sketch3 (4)" against normal blind 1.1 contours L2 L3 A1 | L1 L2 A1 bodies 30 in component "main-switchbody (5)"
sketch "Sketch4 (4)" plane through (0, 0, 0) normal (0, -1, 0) x (1, 0, 0) in component "main-switchbody (5)"
  line L0 (3.05, 0) -> (6.05, 0)
  line L1 (6.05, 0) -> (6.05, 6)
  line L2 (6.05, 6) -> (3.05, 6)
  line L3 (3.05, 6) -> (3.05, 0)
  line L4 (3.05, 6) -> (3.05, 4.5) construction
  line L5 (6.05, 6) -> (6.05, 4.5) construction
  arc A0 (6.05, 4.5) -> (3.05, 4.5) centre (4.55, 4.5) ccw
  constraint coincident L2.end L3.start
  constraint coincident L3 L4.end
  constraint perpendicular L2 L4
  constraint coincident L1.end L2.start
  constraint coincident L1 L5.end
  constraint perpendicular L2 L5
  constraint tangent L2 A0
extrude "Extrude8'''" cut sketch "Sketch4 (4)" against normal blind 1.1 contours L2 L3 A0 | L1 L2 A0 bodies 29 in component "main-switchbody (5)"
sketch "Sketch5 (4)" plane through (0, 0, 0) normal (0, -1, 0) x (1, 0, 0) in component "main-switchbody (5)"
  line L0 (13.95, 0) -> (16.95, 0)
  line L1 (16.95, 0) -> (16.95, 6)
  line L2 (16.95, 6) -> (13.95, 6)
  line L3 (13.95, 6) -> (13.95, 0)
  line L4 (13.95, 6) -> (13.95, 4.5) construction
  line L5 (16.95, 6) -> (16.95, 4.5) construction
  arc A0 (16.95, 4.5) -> (13.95, 4.5) centre (15.45, 4.5) ccw
  constraint coincident L2.end L3.start
  constraint coincident L3 L4.end
  constraint perpendicular L2 L4
  constraint coincident L1.end L2.start
  constraint coincident L1 L5.end
  constraint perpendicular L2 L5
  constraint tangent L2 A0
extrude "Extrude9'''" cut sketch "Sketch5 (4)" against normal blind 1.1 contours L2 L3 A0 | L1 L2 A0 bodies 31 in component "main-switchbody (5)"
sketch "Sketch6 (4)" plane through (0, 18.9, 0) normal (0, -1, 0) x (1, 0, 0) in component "main-switchbody (5)"
  line L0 (13.95, 0) -> (16.95, 0)
  line L1 (16.95, 0) -> (16.95, 6)
  line L2 (16.95, 6) -> (13.95, 6)
  line L3 (13.95, 6) -> (13.95, 0)
  line L4 (13.95, 6) -> (13.95, 4.5) construction
  line L5 (16.95, 6) -> (16.95, 4.5) construction
  arc A0 (16.95, 4.5) -> (13.95, 4.5) centre (15.45, 4.5) ccw
  constraint coincident L2.end L3.start
  constraint coincident L3 L4.end
  constraint perpendicular L2 L4
  constraint coincident L1.end L2.start
  constraint coincident L1 L5.end
  constraint perpendicular L2 L5
  constraint tangent L2 A0
extrude "Extrude10'''" cut sketch "Sketch6 (4)" against normal blind 1.1 contours L2 L3 A0 | L1 L2 A0 bodies 32 in component "main-switchbody (5)"
sketch "Sketch7 (4)" plane through (0, 0, 4) normal (0, 0, 1) x (-1, 0, 0) in component "main-switchbody (5)"
  line L0 (-3.05, -16.95) -> (-16.95, -16.95)
  line L1 (-16.95, -16.95) -> (-16.95, -3.05)
  line L2 (-16.95, -3.05) -> (-3.05, -3.05)
  line L3 (-3.05, -3.05) -> (-3.05, -16.95)
  line L4 (-6.05, -20) -> (-6.05, -18.9)
  line L5 (-6.05, -18.9) -> (-3.05, -18.9)
  line L6 (-3.05, -18.9) -> (-3.05, -20)
  line L7 (-3.05, -20) -> (0, -20)
  line L8 (0, -20) -> (0, 0)
  line L9 (0, 0) -> (-3.05, 0)
  line L10 (-3.05, 0) -> (-3.05, -1.1)
  line L11 (-3.05, -1.1) -> (-6.05, -1.1)
  line L12 (-6.05, -1.1) -> (-6.05, 0)
  line L13 (-6.05, 0) -> (-13.95, 0)
  line L14 (-13.95, 0) -> (-13.95, -1.1)
  line L15 (-13.95, -1.1) -> (-16.95, -1.1)
  line L16 (-16.95, -1.1) -> (-16.95, 0)
  line L17 (-16.95, 0) -> (-20, 0)
  line L18 (-20, 0) -> (-20, -20)
  line L19 (-20, -20) -> (-16.95, -20)
  line L20 (-16.95, -20) -> (-16.95, -18.9)
  line L21 (-16.95, -18.9) -> (-13.95, -18.9)
  line L22 (-13.95, -18.9) -> (-13.95, -20)
  line L23 (-13.95, -20) -> (-6.05, -20)
  line L24 (-20, -10) -> (-20, -11.5) construction
  line L25 (-20, -10) -> (-20, -8.5) construction
  line L26 (-20, -8.5) -> (-19, -8.5) construction
  line L27 (-19, -8.5) -> (-19, -11.5) construction
  line L28 (-19, -11.5) -> (-20, -11.5) construction
  line L29 (-20, -11.5) -> (-21, -11.5) construction
  line L30 (-21, -11.5) -> (-21, -8.5) construction
  line L31 (-21, -8.5) -> (-20, -8.5) construction
  line L32 (-19, -11.5) -> (-21, -11.5)
  line L33 (-21, -11.5) -> (-21, -8.5)
  line L34 (-21, -8.5) -> (-19, -8.5)
  line L35 (-19, -8.5) -> (-19, -11.5)
  dimension "d41_9" = 1.5
  dimension "d42_9" = 1
  constraint midpoint L18 L24.start
  constraint parallel L18 L24
  constraint coincident L18 L25.end
  constraint parallel L18 L25
  constraint perpendicular L25 L26
  constraint perpendicular L26 L27
  constraint perpendicular L24 L29
  constraint perpendicular L29 L30
  constraint horizontal L32
  constraint vertical L33
  constraint horizontal L34
  constraint vertical L35
  measures "d41_9" distance of L24.start L24.end
  measures "d42_9" distance of L24.end L29.end
extrude "Extrude11'''" add sketch "Sketch7 (4)" along normal blind 3 contours L18 L32 L33 L34 | L18 L32 L34 L35 bodies 28 in component "main-switchbody (5)"
extrude "Extrude12'''" add 1 faces at (20, 8.5, 6) along direction (0, -1, 0) blind 0.5 on bodies 28 bodies 28 in component "main-switchbody (5)"
extrude "Extrude13'''" add 1 faces at (20, 11.5, 6) along direction (0, 1, 0) blind 0.5 on bodies 28 bodies 28 in component "main-switchbody (5)"
extrude "Extrude14'''" add 1 faces at (20.3333, 10.6667, 7) along direction (0, 0, 1) blind 0.75 on bodies 28 bodies 28 in component "main-switchbody (5)"
sketch "Sketch8 (4)" plane through (0, 0, 4) normal (0, 0, -1) x (1, 0, 0) in component "main-switchbody (5)"
  line L0 (20, -8) -> (20, -12)
  line L1 (20, -12) -> (21, -12)
  line L2 (21, -12) -> (21, -8)
  line L3 (21, -8) -> (20, -8)
  line L4 (20, -12) -> (20, -8)
  constraint coincident L0.end L1.start
  constraint coincident L0.start L3.end
extrude "Extrude15'''" add sketch "Sketch8 (4)" along normal blind 2 bodies 28 in component "main-switchbody (5)"
sketch "Sketch9 (7)" plane through (19, 0, 0) normal (-1, 0, 0) x (0, -1, 0) in component "main-switchbody (5)"
  line L0 (-12, 4) -> (-8, 4)
  line L1 (-8, 4) -> (-8, 7.75)
  line L2 (-8, 7.75) -> (-12, 7.75)
  line L3 (-12, 7.75) -> (-12, 4)
  line L4 (-12, 7.75) -> (-12, 5.75) construction
  line L5 (-12, 5.75) -> (-8, 5.75) construction
  line L6 (-12, 7.75) -> (-8, 7.75)
  line L7 (-8, 7.75) -> (-8, 5.75)
  line L8 (-8, 5.75) -> (-12, 5.75)
  line L9 (-12, 5.75) -> (-12, 7.75)
  dimension "d53_9" = 2
  constraint coincident L2.end L3.start
  constraint perpendicular L2 L4
  constraint coincident L1 L5.end
  constraint perpendicular L1 L5
  constraint horizontal L6
  constraint vertical L7
  constraint horizontal L8
  constraint vertical L9
  measures "d53_9" distance of L2.end L4.end
extrude "Extrude16'''" add sketch "Sketch9 (7)" along normal blind 0.5 contours L1 L2 L3 L6 L7 L8 L9 bodies 28 in component "main-switchbody (5)"
extrude "Extrude17'''" cut 1 faces at (2.1, 9.3333, 6.9167) along direction (-1, 0, 0) blind 0.3 on bodies 27 bodies 27 in component "main-switchbody (5)"
extrude "Extrude18'''" cut sketch "Sketch1 (18)" along normal blind 2.7 contours L44 L84 L85 L86 L87 bodies 28 in component "main-switchbody (5)"
extrude "Extrude19'''" cut sketch "Sketch1 (18)" along normal blind 2.7 contours L46 L80 L81 L82 L83 bodies 28 in component "main-switchbody (5)"
extrude "Extrude20'''" add sketch "Sketch1 (18)" against normal blind 0.2 contours L39 L40 L41 L42 L47 L48 L50 L51 L52 L54 L56 L57 L58 L60 L61 L62 L63 L64 L65 L66 L67 L68 | L39 L59 L60 L61 L62 | L42 L63 L64 L65 L66 L67 L68 | L39 L55 L56 L57 L58 | L41 L47 L48 L49 L50 | L41 L51 L52 L53 L54 bodies 27 28 29 30 31 32 in component "main-switchbody (5)"
fillet "Fillet1'''" radius 1 2 edges at (21, 10, 7.75) (-0.9, 10, 7.5) on bodies 27 28 in component "main-switchbody (5)"
extrude "Extrude21'''" add 1 faces at (2.8833, 9.1667, 2.7) along direction (0, 0, -1) blind 2.9 on bodies 27 bodies 27 in component "main-switchbody (5)"
extrude "Extrude22'''" add 1 faces at (17.1167, 10.8333, 2.7) along direction (0, 0, -1) blind 2.9 on bodies 27 bodies 27 in component "main-switchbody (5)"
sketch "Sketch10 (4)" plane through (0, 0, 4) normal (0, 0, 1) x (-1, 0, 0) in component "main-switchbody (5)"
  line L0 (-3.05, -16.95) -> (-16.95, -16.95)
  line L1 (-16.95, -16.95) -> (-16.95, -3.05)
  line L2 (-16.95, -3.05) -> (-3.05, -3.05)
  line L3 (-3.05, -3.05) -> (-3.05, -16.95)
  line L4 (0, -12) -> (-1.1, -12)
  line L5 (-1.1, -12) -> (-1.1, -8)
  line L6 (-1.1, -8) -> (0, -8)
  line L7 (0, -8) -> (0, 0)
  line L8 (0, 0) -> (-3.05, 0)
  line L9 (-3.05, 0) -> (-3.05, -1.1)
  line L10 (-3.05, -1.1) -> (-6.05, -1.1)
  line L11 (-6.05, -1.1) -> (-6.05, 0)
  line L12 (-6.05, 0) -> (-13.95, 0)
  line L13 (-13.95, 0) -> (-13.95, -1.1)
  line L14 (-13.95, -1.1) -> (-16.95, -1.1)
  line L15 (-16.95, -1.1) -> (-16.95, 0)
  line L16 (-16.95, 0) -> (-20, 0)
  line L17 (-20, 0) -> (-20, -8)
  line L18 (-20, -8) -> (-19, -8)
  line L19 (-19, -8) -> (-19, -12)
  line L20 (-19, -12) -> (-20, -12)
  line L21 (-20, -12) -> (-20, -20)
  line L22 (-20, -20) -> (-16.95, -20)
  line L23 (-16.95, -20) -> (-16.95, -18.9)
  line L24 (-16.95, -18.9) -> (-13.95, -18.9)
  line L25 (-13.95, -18.9) -> (-13.95, -20)
  line L26 (-13.95, -20) -> (-6.05, -20)
  line L27 (-6.05, -20) -> (-6.05, -18.9)
  line L28 (-6.05, -18.9) -> (-3.05, -18.9)
  line L29 (-3.05, -18.9) -> (-3.05, -20)
  line L30 (-3.05, -20) -> (0, -20)
  line L31 (0, -20) -> (0, -12)
  line L32 (-3.05, -10) -> (-3.05, -12.5) construction
  line L33 (-3.05, -12.5) -> (-3.05, -7.5) construction
  line L34 (-3.05, -7.5) -> (-2.55, -7.5) construction
  line L35 (-2.55, -7.5) -> (-3.05, -7.5) construction
  line L36 (-3.05, -7.5) -> (-3.05, -12.5) construction
  line L37 (-3.05, -12.5) -> (-2.55, -12.5) construction
  line L38 (-2.55, -12.5) -> (-2.55, -7.5) construction
  line L39 (-3.05, -12.5) -> (-16.95, -12.5) construction
  line L40 (-16.95, -12.5) -> (-16.95, -7.5) construction
  line L41 (-16.95, -7.5) -> (-17.45, -7.5) construction
  line L42 (-17.45, -7.5) -> (-16.95, -7.5) construction
  line L43 (-16.95, -7.5) -> (-16.95, -12.5) construction
  line L44 (-16.95, -12.5) -> (-17.45, -12.5) construction
  line L45 (-17.45, -12.5) -> (-17.45, -7.5) construction
  line L46 (-16.95, -12.5) -> (-17.45, -12.5)
  line L47 (-17.45, -12.5) -> (-17.45, -7.5)
  line L48 (-17.45, -7.5) -> (-16.95, -7.5)
  line L49 (-16.95, -7.5) -> (-16.95, -12.5)
  line L50 (-2.55, -12.5) -> (-3.05, -12.5)
  line L51 (-3.05, -12.5) -> (-3.05, -7.5)
  line L52 (-3.05, -7.5) -> (-2.55, -7.5)
  line L53 (-2.55, -7.5) -> (-2.55, -12.5)
  dimension "d75_5" = 5
  dimension "d76_5" = 0.5
  dimension "d77_5" = 0.5
  constraint midpoint L3 L32.start
  constraint coincident L3 L32.end
  constraint perpendicular L0 L32
  constraint parallel L3 L33
  constraint perpendicular L33 L34
  constraint horizontal L35
  constraint vertical L36
  constraint horizontal L37
  constraint vertical L38
  constraint coincident L1 L39.end
  constraint perpendicular L1 L39
  constraint coincident L1 L40.end
  constraint perpendicular L39 L40
  constraint perpendicular L40 L41
  constraint horizontal L42
  constraint vertical L43
  constraint horizontal L44
  constraint vertical L45
  constraint horizontal L46
  constraint vertical L47
  constraint horizontal L48
  constraint vertical L49
  constraint horizontal L50
  constraint vertical L51
  constraint horizontal L52
  constraint vertical L53
  measures "d75_5" distance of L32.end L33.end
  measures "d76_5" distance of L33.end L34.end
  measures "d77_5" distance of L40.end L41.end
extrude "Extrude23'''" cut sketch "Sketch10 (4)" against normal blind 2.9 contours L3 L50 L51 L52 L53 | L1 L46 L47 L48 L49 bodies 27 in component "main-switchbody (5)"
extrude "Extrude24'''" cut 2 faces at (4.8122, 18.9, 5.1079) (15.1626, 18.9, 5.4316) along direction (0, 1, 0) blind 0.25 on bodies 27 bodies 27 in component "main-switchbody (5)"
extrude "Extrude25'''" cut 2 faces at (4.2822, 1.1, 5.1824) (15.2673, 1.1, 4.9654) along direction (0, -1, 0) blind 0.25 on bodies 27 bodies 27 in component "main-switchbody (5)"
extrude "Extrude26'''" add 1 faces at (1.0167, 12.3167, -0.2) along direction (0, 0, -1) blind 1 on bodies 27 bodies 27 in component "main-switchbody (5)"
extrude "Extrude27'''" cut 1 faces at (1.0167, 12.3167, -1.2) along direction (0, 0, 1) blind 0.2 on bodies 27 bodies 27 in component "main-switchbody (5)"
extrude "Extrude28'''" cut 2 faces at (17.1167, 10.8333, 1.1) (2.8833, 9.1667, 1.1) along direction (0, 0, -1) blind 0.8 on bodies 27 bodies 27 in component "main-switchbody (5)"
extrude "Extrude29'''" cut 1 faces at (18.8333, 9.3333, 5.75) along direction (0, 0, 1) blind 0.2 on bodies 27 bodies 27 in component "main-switchbody (5)"
extrude "Extrude30'''" cut 1 faces at (1.3333, 10.6667, 5.75) along direction (0, 0, 1) blind 0.2 on bodies 27 bodies 27 in component "main-switchbody (5)"
sketch "Sketch1 (19)" plane through (0, 0, 0.0152) normal (0, 0, -1) x (1, 0, 0) in component "mxledbit-switchbody v10 (5)"
  line L0 (4.5419, -16.2374) -> (4.5419, -2.3374)
  line L1 (4.5419, -2.3374) -> (18.4419, -2.3374)
  line L2 (18.4419, -2.3374) -> (18.4419, -16.2374)
  line L3 (18.4419, -16.2374) -> (4.5419, -16.2374)
  line L4 (1.4919, -19.2874) -> (21.4919, -19.2874)
  line L5 (21.4919, -19.2874) -> (21.4919, 0.7126)
  line L6 (21.4919, 0.7126) -> (1.4919, 0.7126)
  line L7 (1.4919, 0.7126) -> (1.4919, -19.2874)
ref_plane "WorkPlane1" through (5, 51, 10) normal (0, -1, 0) x (1, 0, 0) in component "wheel (3)"
sketch "Sketch2 (15)" plane through (5, 51, 10) normal (0, -1, 0) x (1, 0, 0) in component "wheel (3)"
  circle A0 centre (0, 0) radius 75
  dimension "d64_7" = 150
  constraint coincident A0.centre origin
  measures "d64_7" diameter of A0
component_pattern "component pattern'''" in component "Ring"
sketch "Sketch2 (16)" plane through (0, 49, 0) normal (0, -1, 0) x (1, 0, 0) in component "IND-Sketch (3)"
  circle A0 centre (5, 10) radius 75
  line L0 (5, 10) -> (5, -65) construction
  line L1 (5, -65) -> (-19.5, -65) construction
  line L2 (-19.5, -65) -> (29.5, -65)
  line L3 (29.5, -65) -> (29.5, 10)
  line L4 (29.5, 10) -> (-19.5, 10)
  line L5 (-19.5, 10) -> (-19.5, -65)
  dimension "d69_7" = 75
  dimension "d70_7" = 24.5
  dimension "d71_7" = 49
  dimension "d72_7" = 75
  constraint coincident A0.centre L0.start
  constraint vertical L0
  constraint perpendicular L0 L1
  constraint horizontal L2
  constraint vertical L3
  constraint horizontal L4
  constraint vertical L5
  measures "d69_7" distance of A0.centre L0.end
  measures "d70_7" distance of L0.end L1.end
  measures "d71_7" distance of L1.end L2.end
  measures "d72_7" distance of L1.end L4.end
sketch "Sketch9 (8)" plane through (5, 41.9534, 55.6343) normal (0, 0.573576, 0.819152) x (-1, 0, 0) in component "IND-Sketch (3)"
  line L0 (-45, -9.823) -> (5, -9.823) construction
  line L1 (-20, -9.823) -> (5, -9.823) construction
  line L2 (-20, -9.823) -> (-45, -9.823) construction
  circle A0 centre (-20, -9.823) radius 75 construction
  point P0 (-20, -9.823)
  point P1 (-45, -9.823)
  point P2 (5, -9.823)
  point P3 (5, -9.823)
  point P4 (-45, -9.823)
  dimension "d38_7" = 49
  dimension "d39_7" = 24.5
  dimension "d40_7" = 24.5
  dimension "d41_7" = 150
  constraint coincident P4 P1
  constraint horizontal L0
  constraint coincident P0 L1.start
  constraint parallel L0 L1
  constraint parallel L0 L2
  measures "d41_7" diameter of A0
sketch "Sketch1 (20)" plane through (0, 54.7581, -45.9475) normal (0, -0.766044, 0.642788) x (1, 0, 0) in component "IND-Sketch (3)"
  line L0 (-1.3269, 70.632) -> (-1.3269, 84.532)
  line L1 (-1.3269, 84.532) -> (12.5731, 84.532)
  line L2 (12.5731, 84.532) -> (12.5731, 70.632)
  line L3 (12.5731, 70.632) -> (-1.3269, 70.632)
  line L4 (-4.3769, 67.582) -> (15.6231, 67.582)
  line L5 (15.6231, 67.582) -> (15.6231, 87.582)
  line L6 (15.6231, 87.582) -> (-4.3769, 87.582)
  line L7 (-4.3769, 87.582) -> (-4.3769, 67.582)
  line L8 (-4.3769, 77.582) -> (15.6231, 77.582) construction
  line L9 (5.6231, 87.582) -> (5.6231, 67.582) construction
  point P0 (5.6231, 77.582)
  constraint midpoint L7 L8.start
  constraint midpoint L5 L8.end
  constraint midpoint L6 L9.start
  constraint midpoint L4 L9.end
  constraint midpoint L8 P0
ref_plane "WorkPlane2" through (0, 65, 0) normal (0, 1, 0) x (0, 0, 1) in component "IND-Sketch (4)"